Autodesk Fusion 360 part; units mm, degrees
(part 2 of 3)
sketch "Boceto7" plane through (1067.9423, 0, 0) normal (1, 0, 0) x (0, 0, -1)
  line L0 (-357.5, 27) -> (-357.5, -50.5)
  line L1 (-292.5, -50.5) -> (-292.5, 27)
  line L2 (-297.5, 22) -> (-352.5, 22)
  line L3 (-352.5, 22) -> (-352.5, -45.5)
  line L4 (-352.5, -45.5) -> (-297.5, -45.5)
  line L5 (-297.5, -11.75) -> (-352.5, -11.75) construction
  line L6 (-332.5, -16.0801) -> (-325, -20.4103)
  line L7 (-325, -20.4103) -> (-317.5, -16.0801)
  line L8 (-317.5, -16.0801) -> (-317.5, -7.4199)
  line L9 (-317.5, -7.4199) -> (-325, -3.0897)
  line L10 (-325, -3.0897) -> (-332.5, -7.4199)
  line L11 (-332.5, -7.4199) -> (-332.5, -16.0801)
  line L12 (-325, -11.75) -> (-328.75, -18.2452) construction
  line L13 (-297.5, 12.7874) -> (-302.5, 9.9006)
  line L14 (-302.5, 9.9006) -> (-302.5, 1.2404)
  line L15 (-302.5, 1.2404) -> (-297.5, -1.6464)
  line L16 (-297.5, -7.4199) -> (-305, -3.0897)
  line L17 (-305, -3.0897) -> (-312.5, -7.4199)
  line L18 (-312.5, -7.4199) -> (-312.5, -16.0801)
  line L19 (-312.5, -16.0801) -> (-305, -20.4103)
  line L20 (-305, -20.4103) -> (-297.5, -16.0801)
  line L21 (-312.5, 22) -> (-312.5, 18.5609)
  line L22 (-312.5, 18.5609) -> (-305, 14.2308)
  line L23 (-297.5, 18.5609) -> (-297.5, 22)
  line L24 (-305, 14.2308) -> (-297.5, 18.5609)
  line L25 (-307.5, 9.9006) -> (-315, 14.2308)
  line L26 (-315, 14.2308) -> (-322.5, 9.9006)
  line L27 (-322.5, 9.9006) -> (-322.5, 1.2404)
  line L28 (-322.5, 1.2404) -> (-315, -3.0897)
  line L29 (-307.5, 1.2404) -> (-307.5, 9.9006)
  line L30 (-315, -3.0897) -> (-307.5, 1.2404)
  line L31 (-332.5, 22) -> (-332.5, 18.5609)
  line L32 (-332.5, 18.5609) -> (-325, 14.2308)
  line L33 (-317.5, 18.5609) -> (-317.5, 22)
  line L34 (-325, 14.2308) -> (-317.5, 18.5609)
  line L35 (-327.5, 9.9006) -> (-335, 14.2308)
  line L36 (-335, 14.2308) -> (-342.5, 9.9006)
  line L37 (-342.5, 9.9006) -> (-342.5, 1.2404)
  line L38 (-342.5, 1.2404) -> (-335, -3.0897)
  line L39 (-327.5, 1.2404) -> (-327.5, 9.9006)
  line L40 (-335, -3.0897) -> (-327.5, 1.2404)
  line L41 (-337.5, -7.4199) -> (-345, -3.0897)
  line L42 (-345, -3.0897) -> (-352.5, -7.4199)
  line L43 (-352.5, -7.4199) -> (-352.5, -16.0801)
  line L44 (-352.5, -16.0801) -> (-345, -20.4103)
  line L45 (-337.5, -16.0801) -> (-337.5, -7.4199)
  line L46 (-345, -20.4103) -> (-337.5, -16.0801)
  line L47 (-352.5, 22) -> (-352.5, 18.5609)
  line L48 (-352.5, 18.5609) -> (-345, 14.2308)
  line L49 (-337.5, 18.5609) -> (-337.5, 22)
  line L50 (-345, 14.2308) -> (-337.5, 18.5609)
  line L51 (-347.5, 9.9006) -> (-352.5, 12.7874)
  line L52 (-347.5, 1.2404) -> (-347.5, 9.9006)
  line L53 (-352.5, -1.6464) -> (-347.5, 1.2404)
  line L54 (-297.5, -21.8536) -> (-302.5, -24.7404)
  line L55 (-302.5, -24.7404) -> (-302.5, -33.4006)
  line L56 (-297.5, -42.0609) -> (-305, -37.7308)
  line L57 (-305, -37.7308) -> (-312.5, -42.0609)
  line L58 (-312.5, -42.0609) -> (-312.5, -45.5)
  line L59 (-297.5, -45.5) -> (-297.5, -42.0609)
  line L60 (-307.5, -24.7404) -> (-315, -20.4103)
  line L61 (-315, -20.4103) -> (-322.5, -24.7404)
  line L62 (-322.5, -24.7404) -> (-322.5, -33.4006)
  line L63 (-322.5, -33.4006) -> (-315, -37.7308)
  line L64 (-307.5, -33.4006) -> (-307.5, -24.7404)
  line L65 (-315, -37.7308) -> (-307.5, -33.4006)
  line L66 (-317.5, -42.0609) -> (-325, -37.7308)
  line L67 (-325, -37.7308) -> (-332.5, -42.0609)
  line L68 (-332.5, -42.0609) -> (-332.5, -45.5)
  line L69 (-317.5, -45.5) -> (-317.5, -42.0609)
  line L70 (-327.5, -24.7404) -> (-335, -20.4103)
  line L71 (-335, -20.4103) -> (-342.5, -24.7404)
  line L72 (-342.5, -24.7404) -> (-342.5, -33.4006)
  line L73 (-342.5, -33.4006) -> (-335, -37.7308)
  line L74 (-327.5, -33.4006) -> (-327.5, -24.7404)
  line L75 (-335, -37.7308) -> (-327.5, -33.4006)
  line L76 (-337.5, -42.0609) -> (-345, -37.7308)
  line L77 (-345, -37.7308) -> (-352.5, -42.0609)
  line L78 (-352.5, -42.0609) -> (-352.5, -45.5)
  line L79 (-337.5, -45.5) -> (-337.5, -42.0609)
  line L80 (-347.5, -24.7404) -> (-352.5, -21.8536)
  line L81 (-347.5, -33.4006) -> (-347.5, -24.7404)
  line L82 (-352.5, -36.2874) -> (-347.5, -33.4006)
  line L83 (-297.5, -45.5) -> (-297.5, -42.0609)
  line L84 (-297.5, 18.5609) -> (-297.5, 22)
  line L85 (-297.5, -45.5) -> (-297.5, 22)
  line L86 (-325, -20.4103) -> (-325, -3.0897) construction
  line L87 (-297.5, -36.2874) -> (-302.5, -33.4006)
  point P0 (-325, -11.75)
  dimension "d33" = 7.5
  constraint midpoint L3 L5.end
  constraint midpoint L5 P0
  constraint parallel L3 L11
  constraint coincident P0 L12.start
  constraint midpoint L6 L12.end
  constraint coincident L4 L58.end
  constraint coincident L4 L69.start
  constraint coincident L4 L68.end
  constraint coincident L4 L79.start
  constraint coincident L3 L82.start
  constraint coincident L3 L80.end
  constraint coincident L3 L53.start
  constraint coincident L3 L51.end
  constraint coincident L2 L49.end
  constraint coincident L2 L31.start
  constraint coincident L2 L33.end
  constraint coincident L2 L21.start
  constraint collinear L83 L84
  constraint perpendicular L2 L85
  constraint symmetric L81.start L86 L55.end
  constraint symmetric L82.start L86 L87.start
  measures "d33" distance of P0 L11
extrude "Extruir5" cut sketch "Boceto7" against normal blind 240 contours L2 L21 L22 L23 L24 L84 L85 | L2 L31 L32 L33 L34 | L13 L14 L15 L85 | L2 L3 L47 L48 L49 L50 | L16 L17 L18 L19 L20 L85 | L54 L55 L85 L87 | L3 L51 L52 L53 | L4 L56 L57 L58 L59 L83 L85 | L3 L41 L42 L43 L44 L45 L46 | L3 L80 L81 L82 | L4 L66 L67 L68 L69 | L3 L4 L76 L77 L78 L79 | L6 L7 L8 L9 L10 L11 | L25 L26 L27 L28 L29 L30 | L35 L36 L37 L38 L39 L40 | L60 L61 L62 L63 L64 L65 | L70 L71 L72 L73 L74 L75 bodies 2 3
move_body "Desplazar1" bodies 1 2 3 to x (1, 0, 0) y (0, 1, 0) z (0, 0, 1) at (-888.5759, -26.6129, 0)
sketch "Boceto9" plane through (0, 0, 292.5) normal (0, 0, -1) x (-1, 0, 0)
  line L0 (0.6336, 0.3871) -> (-2.3664, 0.3871)
  line L1 (-2.3664, 0.3871) -> (-2.3664, -77.1129)
  line L2 (-2.3664, -77.1129) -> (0.6336, -77.1129)
  line L3 (0.6336, -77.1129) -> (0.6336, 0.3871)
  line L4 (0.6336, -77.1129) -> (-41.8664, -77.1129) construction
  line L5 (-41.8664, -77.1129) -> (-41.8664, -119.6129) construction
  arc A0 (-37.7625, -116.3992) -> (-2.5802, -81.2168) centre (-41.8664, -77.1129) ccw
  arc A1 (-41.8664, -119.6129) -> (0.6336, -77.1129) centre (-41.8664, -77.1129) ccw
  line L6 (0.6336, 0.3871) -> (-179.3664, 0.3871)
  line L7 (-89.3664, 0.3871) -> (-89.3664, -20) construction
  line L8 (-41.8664, -116.6129) -> (-41.8664, -119.6129)
  line L9 (0.6336, -77.1129) -> (-2.3664, -77.1129)
  line L10 (-2.3664, -77.1129) -> (-2.3664, -70.1129)
  line L11 (-2.3664, -70.1129) -> (-5.3664, -70.1129)
  line L12 (-5.3664, -70.1129) -> (-5.3664, -80.1129)
  line L13 (-5.3664, -80.1129) -> (-3.5748, -80.1129)
  line L14 (-41.8664, -116.6129) -> (-48.8664, -116.6129)
  line L15 (-48.8664, -116.6129) -> (-48.8664, -113.6129)
  line L16 (-48.8664, -113.6129) -> (-38.8664, -113.6129)
  line L17 (-38.8664, -113.6129) -> (-38.8664, -115.4046)
  arc A2 (-2.5802, -81.2168) -> (-3.5748, -80.1129) centre (-3.5748, -81.1129) ccw
  arc A3 (-38.8664, -115.4046) -> (-37.7625, -116.3992) centre (-37.8664, -115.4046) ccw
  arc A4 (-179.3664, -77.1129) -> (-136.8664, -119.6129) centre (-136.8664, -77.1129) ccw
  line L18 (-129.8664, -116.6129) -> (-129.8664, -113.6129)
  arc A5 (-176.1526, -81.2168) -> (-140.9703, -116.3992) centre (-136.8664, -77.1129) ccw
  line L19 (-136.8664, -77.1129) -> (-136.8664, -119.6129) construction
  line L20 (-136.8664, -116.6129) -> (-129.8664, -116.6129)
  arc A6 (-140.9703, -116.3992) -> (-139.8664, -115.4046) centre (-140.8664, -115.4046) ccw
  line L21 (-176.3664, -77.1129) -> (-176.3664, -70.1129)
  line L22 (-173.3664, -70.1129) -> (-173.3664, -80.1129)
  line L23 (-179.3664, -77.1129) -> (-176.3664, -77.1129)
  line L24 (-129.8664, -113.6129) -> (-139.8664, -113.6129)
  line L25 (-136.8664, -116.6129) -> (-136.8664, -119.6129)
  line L26 (-179.3664, -77.1129) -> (-136.8664, -77.1129) construction
  line L27 (-176.3664, -70.1129) -> (-173.3664, -70.1129)
  line L28 (-176.3664, -77.1129) -> (-179.3664, -77.1129)
  line L29 (-173.3664, -80.1129) -> (-175.158, -80.1129)
  line L30 (-139.8664, -113.6129) -> (-139.8664, -115.4046)
  arc A7 (-175.158, -80.1129) -> (-176.1526, -81.2168) centre (-175.158, -81.1129) ccw
  dimension "d40" = 42.5
  dimension "d41" = 42.5
  dimension "d44" = 7
  dimension "d45" = 3
  dimension "d46" = 10
  dimension "d47" = 7
  dimension "d48" = 3
  dimension "d49" = 10
  dimension "d50" = 1
  dimension "d51" = 1
  constraint coincident L2.end L3.start
  constraint perpendicular L3 L4
  constraint vertical L5
  constraint coincident L4.end L5.start
  constraint concentric A0 A1
  constraint coincident L5 L8.start
  constraint midpoint L6 L7.start
  constraint perpendicular L6 L7
  constraint coincident L1.end L2.start
  constraint perpendicular L4 L10
  constraint perpendicular L10 L11
  constraint perpendicular L11 L12
  constraint perpendicular L12 L13
  constraint perpendicular L5 L14
  constraint perpendicular L14 L15
  constraint perpendicular L15 L16
  constraint perpendicular L16 L17
  constraint tangent A0 A2
  constraint tangent L13 A2
  constraint tangent A0 A3
  constraint tangent L17 A3
  constraint symmetric L1.end L7 L21.start
  constraint symmetric L2.end L7 A4.start
  constraint symmetric L4.end L7 A4.centre
  constraint symmetric L5.end L7 A4.end
  constraint symmetric L8.start L7 L20.start
  constraint symmetric A0 L7 A5
  constraint symmetric A1 L7 A4
  constraint symmetric L7 L1.end L21.start
  constraint symmetric L7 L10.end L21.end
  constraint symmetric L7 L11.end L22.start
  constraint symmetric L7 L12.end L22.end
  constraint symmetric L7 L14.end L18.start
  constraint symmetric L7 L15.end L18.end
  constraint symmetric L7 L16.end L24.end
  constraint symmetric L7 L13.end L29.end
  constraint symmetric L7 A0.end A5.start
  constraint symmetric L7 A2 A7
  constraint symmetric L7 L17.end A6.end
  constraint symmetric L7 A0.start A5.end
  constraint symmetric L7 A3 A6
  measures "d40" distance of L2.end L4.end
  measures "d41" distance of L4.end L5.end
  measures "d44" distance of L1.end L10.end
  measures "d45" distance of L10.end L11.end
  measures "d46" distance of L11.end L12.end
  measures "d47" distance of L8.start L14.end
  measures "d48" distance of L14.end L15.end
  measures "d49" distance of L15.end L16.end
  measures "d50" radius of A2
  measures "d51" radius of A3
extrude "Extruir6" add sketch "Boceto9" against normal blind 65 separate body contours L1 L2 A0 A1 L8 L9 L10 L11 L12 L13 L14 L15 L16 L17 A2 A3 | A4 L18 A5 L20 A6 L21 L22 L23 L24 L25 L27 L28 L29 L30 A7 makes body 4 at (-0.5855, -79.1352, 335.8333) makes body 5 at (173.6725, -98.3629, 335.8333)
sketch "Boceto10" plane through (0, -116.6129, 0) normal (0, -1, 0) x (1, 0, 0)
  line L0 (129.8664, 292.5) -> (136.8664, 292.5)
  line L1 (136.8664, 292.5) -> (136.8664, 357.5)
  line L2 (136.8664, 357.5) -> (129.8664, 357.5)
  line L3 (41.8664, 292.5) -> (41.8664, 357.5)
  line L4 (136.8664, 292.5) -> (136.8664, 357.5)
  line L5 (41.8664, 357.5) -> (136.8664, 357.5)
  line L6 (136.8664, 357.5) -> (136.8664, 292.5)
  line L7 (136.8664, 292.5) -> (41.8664, 292.5)
  line L8 (41.8664, 292.5) -> (41.8664, 357.5)
  constraint horizontal L5
  constraint vertical L6
  constraint horizontal L7
  constraint vertical L8
  constraint coincident L0.end L1.start
  constraint coincident L3.end L5.start
extrude "Extruir7" add sketch "Boceto10" along normal blind 3 separate body makes body 6
sketch "Boceto11" plane through (0, -119.6129, 0) normal (0, -1, 0) x (1, 0, 0)
  line L0 (136.8664, 292.5) -> (136.8664, 357.5)
  line L1 (136.8664, 357.5) -> (41.8664, 357.5)
  line L2 (41.8664, 357.5) -> (41.8664, 292.5)
  line L3 (46.8664, 297.5) -> (131.8664, 297.5)
  line L4 (131.8664, 352.5) -> (46.8664, 352.5)
  line L5 (46.8664, 352.5) -> (46.8664, 297.5)
  line L6 (46.8664, 325) -> (131.8664, 325) construction
  line L7 (98.0267, 325) -> (93.6965, 332.5)
  line L8 (93.6965, 332.5) -> (85.0363, 332.5)
  line L9 (85.0363, 332.5) -> (80.7061, 325)
  line L10 (80.7061, 325) -> (85.0363, 317.5)
  line L11 (85.0363, 317.5) -> (93.6965, 317.5)
  line L12 (93.6965, 317.5) -> (98.0267, 325)
  line L13 (89.3664, 325) -> (89.3664, 332.5) construction
  line L14 (89.3664, 325) -> (95.8616, 328.75) construction
  line L15 (50.3953, 297.5) -> (59.0555, 297.5)
  line L16 (59.0555, 297.5) -> (63.3856, 305)
  line L17 (63.3856, 305) -> (59.0555, 312.5)
  line L18 (59.0555, 312.5) -> (50.3953, 312.5)
  line L19 (46.8664, 303.6122) -> (50.3953, 297.5)
  line L20 (50.3953, 312.5) -> (46.8664, 306.3878)
  line L21 (50.3953, 317.5) -> (59.0555, 317.5)
  line L22 (59.0555, 317.5) -> (63.3856, 325)
  line L23 (63.3856, 325) -> (59.0555, 332.5)
  line L24 (59.0555, 332.5) -> (50.3953, 332.5)
  line L25 (46.8664, 323.6122) -> (50.3953, 317.5)
  line L26 (50.3953, 332.5) -> (46.8664, 326.3878)
  line L27 (50.3953, 337.5) -> (59.0555, 337.5)
  line L28 (59.0555, 337.5) -> (63.3856, 345)
  line L29 (63.3856, 345) -> (59.0555, 352.5)
  line L30 (59.0555, 352.5) -> (50.3953, 352.5)
  line L31 (46.8664, 343.6122) -> (50.3953, 337.5)
  line L32 (50.3953, 352.5) -> (46.8664, 346.3878)
  line L33 (79.2628, 297.5) -> (76.376, 302.5)
  line L34 (76.376, 302.5) -> (67.7158, 302.5)
  line L35 (67.7158, 302.5) -> (64.829, 297.5)
  line L36 (67.7158, 307.5) -> (76.376, 307.5)
  line L37 (76.376, 307.5) -> (80.7061, 315)
  line L38 (80.7061, 315) -> (76.376, 322.5)
  line L39 (76.376, 322.5) -> (67.7158, 322.5)
  line L40 (63.3856, 315) -> (67.7158, 307.5)
  line L41 (67.7158, 322.5) -> (63.3856, 315)
  line L42 (67.7158, 327.5) -> (76.376, 327.5)
  line L43 (76.376, 327.5) -> (80.7061, 335)
  line L44 (80.7061, 335) -> (76.376, 342.5)
  line L45 (76.376, 342.5) -> (67.7158, 342.5)
  line L46 (63.3856, 335) -> (67.7158, 327.5)
  line L47 (67.7158, 342.5) -> (63.3856, 335)
  line L48 (67.7158, 347.5) -> (76.376, 347.5)
  line L49 (76.376, 347.5) -> (79.2628, 352.5)
  line L50 (64.829, 352.5) -> (67.7158, 347.5)
  line L51 (85.0363, 297.5) -> (93.6965, 297.5)
  line L52 (93.6965, 297.5) -> (98.0267, 305)
  line L53 (98.0267, 305) -> (93.6965, 312.5)
  line L54 (93.6965, 312.5) -> (85.0363, 312.5)
  line L55 (80.7061, 305) -> (85.0363, 297.5)
  line L56 (85.0363, 312.5) -> (80.7061, 305)
  line L57 (85.0363, 337.5) -> (93.6965, 337.5)
  line L58 (93.6965, 337.5) -> (98.0267, 345)
  line L59 (98.0267, 345) -> (93.6965, 352.5)
  line L60 (93.6965, 352.5) -> (85.0363, 352.5)
  line L61 (80.7061, 345) -> (85.0363, 337.5)
  line L62 (85.0363, 352.5) -> (80.7061, 345)
  line L63 (113.9038, 297.5) -> (111.017, 302.5)
  line L64 (111.017, 302.5) -> (102.3568, 302.5)
  line L65 (102.3568, 302.5) -> (99.47, 297.5)
  line L66 (102.3568, 307.5) -> (111.017, 307.5)
  line L67 (111.017, 307.5) -> (115.3472, 315)
  line L68 (115.3472, 315) -> (111.017, 322.5)
  line L69 (111.017, 322.5) -> (102.3568, 322.5)
  line L70 (98.0267, 315) -> (102.3568, 307.5)
  line L71 (102.3568, 322.5) -> (98.0267, 315)
  line L72 (102.3568, 327.5) -> (111.017, 327.5)
  line L73 (111.017, 327.5) -> (115.3472, 335)
  line L74 (115.3472, 335) -> (111.017, 342.5)
  line L75 (111.017, 342.5) -> (102.3568, 342.5)
  line L76 (98.0267, 335) -> (102.3568, 327.5)
  line L77 (102.3568, 342.5) -> (98.0267, 335)
  line L78 (102.3568, 347.5) -> (111.017, 347.5)
  line L79 (111.017, 347.5) -> (113.9038, 352.5)
  line L80 (99.47, 352.5) -> (102.3568, 347.5)
  line L81 (119.6773, 297.5) -> (128.3375, 297.5)
  line L82 (128.3375, 297.5) -> (131.8664, 303.6122)
  line L83 (131.8664, 306.3878) -> (128.3375, 312.5)
  line L84 (128.3375, 312.5) -> (119.6773, 312.5)
  line L85 (115.3472, 305) -> (119.6773, 297.5)
  line L86 (119.6773, 312.5) -> (115.3472, 305)
  line L87 (119.6773, 317.5) -> (128.3375, 317.5)
  line L88 (128.3375, 317.5) -> (131.8664, 323.6122)
  line L89 (131.8664, 326.3878) -> (128.3375, 332.5)
  line L90 (128.3375, 332.5) -> (119.6773, 332.5)
  line L91 (115.3472, 325) -> (119.6773, 317.5)
  line L92 (119.6773, 332.5) -> (115.3472, 325)
  line L93 (119.6773, 337.5) -> (128.3375, 337.5)
  line L94 (128.3375, 337.5) -> (131.8664, 343.6122)
  line L95 (131.8664, 346.3878) -> (128.3375, 352.5)
  line L96 (128.3375, 352.5) -> (119.6773, 352.5)
  line L97 (115.3472, 345) -> (119.6773, 337.5)
  line L98 (119.6773, 352.5) -> (115.3472, 345)
  line L99 (131.8664, 297.5) -> (131.8664, 303.6122)
  line L100 (131.8664, 306.3878) -> (131.8664, 352.5)
  line L101 (131.8664, 303.6122) -> (131.8664, 306.3878)
  point P0 (89.3664, 325)
  dimension "d56" = 15
  constraint midpoint L5 L6.start
  constraint midpoint L6 P0
  constraint parallel L3 L11
  constraint coincident P0 L13.start
  constraint midpoint L8 L13.end
  constraint midpoint L7 L14.end
  constraint coincident L4 L49.end
  constraint coincident L4 L50.start
  constraint coincident L4 L80.start
  constraint coincident L4 L79.end
  constraint coincident L3 L63.start
  constraint coincident L3 L65.end
  constraint coincident L3 L33.start
  constraint coincident L3 L35.end
  constraint coincident L5 L19.start
  constraint coincident L5 L20.end
  constraint coincident L5 L25.start
  constraint coincident L5 L26.end
  constraint coincident L5 L31.start
  constraint coincident L5 L32.end
  constraint coincident L89.start L99
  constraint coincident L88.end L99
  constraint coincident L94.end L99
  constraint coincident L95.start L99
  constraint collinear L99 L100
  constraint coincident L6.end L99
  measures "d56" distance of L8 L11
extrude "Extruir8" cut sketch "Boceto11" against normal blind 20 contours L3 L5 L15 L16 L17 L18 L19 L20 | L3 L33 L34 L35 | L5 L21 L22 L23 L24 L25 L26 | L3 L51 L52 L53 L54 L55 L56 | L4 L5 L27 L28 L29 L30 L31 L32 | L3 L63 L64 L65 | L3 L81 L82 L83 L84 L85 L86 L101 | L4 L48 L49 L50 | L4 L57 L58 L59 L60 L61 L62 | L87 L88 L89 L90 L91 L92 L100 | L4 L78 L79 L80 | L4 L93 L94 L95 L96 L97 L98 L100 | L7 L8 L9 L10 L11 L12 | L36 L37 L38 L39 L40 L41 | L42 L43 L44 L45 L46 L47 | L66 L67 L68 L69 L70 L71 | L72 L73 L74 L75 L76 L77 bodies 6
sketch "Boceto12" plane through (0, 0, 292.5) normal (0, 0, -1) x (-1, 0, 0)
  line L0 (0.6336, 0.3871) -> (-2.3664, 0.3871)
  line L1 (-2.3664, 0.3871) -> (-2.3664, -77.1129)
  line L2 (-2.3664, -77.1129) -> (0.6336, -77.1129)
  line L3 (0.6336, -77.1129) -> (0.6336, 0.3871)
  line L4 (-2.3664, 0.3871) -> (-2.3664, -33.6129)
  line L5 (-2.3664, -33.6129) -> (-176.3664, -33.6129)
  line L6 (-176.3664, -33.6129) -> (-176.3664, -30.6129)
  line L7 (-176.3664, -30.6129) -> (-2.3664, -30.6129)
  line L8 (-2.3664, -30.6129) -> (-2.3664, -33.6129)
  dimension "d63" = 34
  dimension "d64" = 174
  dimension "d65" = 3
  constraint vertical L4
  constraint coincident L0.end L1.start
  constraint horizontal L5
  constraint vertical L6
  constraint horizontal L7
  constraint vertical L8
  measures "d63" distance of L0.end L4.end
  measures "d64" distance of L4.end L5.end
  measures "d65" distance of L4.end L7.end
extrude "Extruir9" add sketch "Boceto12" against normal blind 62 separate body contours L1 L4 L5 L6 L7 L8 makes body 7
sketch "Boceto13" plane through (0, -33.6129, 0) normal (0, -1, 0) x (1, 0, 0)
  line L0 (2.3664, 292.5) -> (176.3664, 292.5)
  line L1 (176.3664, 292.5) -> (176.3664, 354.5)
  line L2 (176.3664, 354.5) -> (2.3664, 354.5)
  line L3 (2.3664, 354.5) -> (2.3664, 292.5)
  line L4 (2.3664, 292.5) -> (176.3664, 292.5)
  line L5 (89.3664, 292.5) -> (136.8664, 292.5)
  line L6 (89.3664, 292.5) -> (41.8664, 292.5)
  line L7 (89.3664, 296.5) -> (41.8664, 296.5)
  line L8 (89.3664, 296.5) -> (136.8664, 296.5)
  line L9 (41.8664, 296.5) -> (136.8664, 296.5)
  line L10 (136.8664, 296.5) -> (136.8664, 300.5)
  line L11 (136.8664, 300.5) -> (41.8664, 300.5)
  line L12 (41.8664, 300.5) -> (41.8664, 296.5)
  dimension "d68" = 47.5
  dimension "d69" = 47.5
  dimension "d70" = 95
  dimension "d71" = 4
  dimension "d72" = 4
  constraint coincident L0.start L3.end
  constraint coincident L0.end L1.start
  constraint midpoint L0 L5.start
  constraint parallel L0 L5
  constraint parallel L4 L6
  constraint horizontal L9
  constraint vertical L10
  constraint horizontal L11
  constraint vertical L12
  measures "d68" distance of L5.start L5.end
  measures "d69" distance of L5.start L6.end
  measures "d70" distance of L5.end L6.end
  measures "d72" distance of L7.end L11.end
extrude "Extruir10" cut sketch "Boceto13" against normal blind 5 contours L7 L8 L9 L10 L11 L12 bodies 7
sketch "Boceto14" plane through (0, 0.3871, 0) normal (0, -1, 0) x (1, 0, 0)
  line L0 (149.9882, 305) -> (154.3183, 312.5)
  line L1 (154.3183, 312.5) -> (162.9786, 312.5)
  line L2 (162.9786, 312.5) -> (167.3087, 305)
  line L3 (167.3087, 305) -> (162.9786, 297.5)
  line L4 (162.9786, 297.5) -> (154.3183, 297.5)
  line L5 (154.3183, 297.5) -> (149.9882, 305)
  line L6 (174.3664, 352.5) -> (174.3664, 347.5)
  line L7 (174.3664, 347.5) -> (171.6388, 347.5)
  line L8 (171.6388, 347.5) -> (168.7521, 352.5)
  line L9 (168.7521, 352.5) -> (174.3664, 352.5)
  line L10 (132.6677, 315) -> (136.9978, 322.5)
  line L11 (136.9978, 322.5) -> (145.6581, 322.5)
  line L12 (145.6581, 322.5) -> (149.9882, 315)
  line L13 (149.9882, 315) -> (145.6581, 307.5)
  line L14 (145.6581, 307.5) -> (136.9978, 307.5)
  line L15 (136.9978, 307.5) -> (132.6677, 315)
  line L16 (115.3472, 345) -> (119.6773, 352.5)
  line L17 (119.6773, 352.5) -> (128.3375, 352.5)
  line L18 (128.3375, 352.5) -> (132.6677, 345)
  line L19 (132.6677, 345) -> (128.3375, 337.5)
  line L20 (128.3375, 337.5) -> (119.6773, 337.5)
  line L21 (119.6773, 337.5) -> (115.3472, 345)
  line L22 (80.7061, 305) -> (85.0363, 312.5)
  line L23 (85.0363, 312.5) -> (93.6965, 312.5)
  line L24 (93.6965, 312.5) -> (98.0267, 305)
  line L25 (98.0267, 305) -> (93.6965, 297.5)
  line L26 (93.6965, 297.5) -> (85.0363, 297.5)
  line L27 (85.0363, 297.5) -> (80.7061, 305)
  line L28 (80.7061, 345) -> (85.0363, 352.5)
  line L29 (85.0363, 352.5) -> (93.6965, 352.5)
  line L30 (93.6965, 352.5) -> (98.0267, 345)
  line L31 (98.0267, 345) -> (93.6965, 337.5)
  line L32 (93.6965, 337.5) -> (85.0363, 337.5)
  line L33 (85.0363, 337.5) -> (80.7061, 345)
  line L34 (46.0651, 325) -> (50.3953, 332.5)
  line L35 (50.3953, 332.5) -> (59.0555, 332.5)
  line L36 (59.0555, 332.5) -> (63.3856, 325)
  line L37 (63.3856, 325) -> (59.0555, 317.5)
  line L38 (59.0555, 317.5) -> (50.3953, 317.5)
  line L39 (50.3953, 317.5) -> (46.0651, 325)
  line L40 (11.4241, 325) -> (15.7542, 332.5)
  line L41 (15.7542, 332.5) -> (24.4145, 332.5)
  line L42 (24.4145, 332.5) -> (28.7446, 325)
  line L43 (28.7446, 325) -> (24.4145, 317.5)
  line L44 (24.4145, 317.5) -> (15.7542, 317.5)
  line L45 (15.7542, 317.5) -> (11.4241, 325)
  line L46 (11.4241, 335) -> (7.094, 327.5)
  line L47 (7.094, 327.5) -> (4.3664, 327.5)
  line L48 (4.3664, 327.5) -> (4.3664, 342.5)
  line L49 (4.3664, 342.5) -> (7.094, 342.5)
  line L50 (7.094, 342.5) -> (11.4241, 335)
  line L51 (11.4241, 345) -> (15.7542, 352.5)
  line L52 (15.7542, 352.5) -> (24.4145, 352.5)
  line L53 (24.4145, 352.5) -> (28.7446, 345)
  line L54 (28.7446, 345) -> (24.4145, 337.5)
  line L55 (24.4145, 337.5) -> (15.7542, 337.5)
  line L56 (15.7542, 337.5) -> (11.4241, 345)
  line L57 (9.9807, 352.5) -> (7.094, 347.5)
  line L58 (7.094, 347.5) -> (4.3664, 347.5)
  line L59 (4.3664, 347.5) -> (4.3664, 352.5)
  line L60 (4.3664, 352.5) -> (9.9807, 352.5)
  line L61 (11.4241, 305) -> (15.7542, 312.5)
  line L62 (15.7542, 312.5) -> (24.4145, 312.5)
  line L63 (24.4145, 312.5) -> (28.7446, 305)
  line L64 (28.7446, 305) -> (24.4145, 297.5)
  line L65 (24.4145, 297.5) -> (15.7542, 297.5)
  line L66 (15.7542, 297.5) -> (11.4241, 305)
  line L67 (46.0651, 305) -> (50.3953, 312.5)
  line L68 (50.3953, 312.5) -> (59.0555, 312.5)
  line L69 (59.0555, 312.5) -> (63.3856, 305)
  line L70 (63.3856, 305) -> (59.0555, 297.5)
  line L71 (59.0555, 297.5) -> (50.3953, 297.5)
  line L72 (50.3953, 297.5) -> (46.0651, 305)
  line L73 (63.3856, 335) -> (67.7158, 342.5)
  line L74 (67.7158, 342.5) -> (76.376, 342.5)
  line L75 (76.376, 342.5) -> (80.7061, 335)
  line L76 (80.7061, 335) -> (76.376, 327.5)
  line L77 (76.376, 327.5) -> (67.7158, 327.5)
  line L78 (67.7158, 327.5) -> (63.3856, 335)
  line L79 (64.829, 297.5) -> (67.7158, 302.5)
  line L80 (67.7158, 302.5) -> (76.376, 302.5)
  line L81 (76.376, 302.5) -> (79.2628, 297.5)
  line L82 (79.2628, 297.5) -> (64.829, 297.5)
  line L83 (99.47, 352.5) -> (113.9038, 352.5)
  line L84 (113.9038, 352.5) -> (111.017, 347.5)
  line L85 (111.017, 347.5) -> (102.3568, 347.5)
  line L86 (102.3568, 347.5) -> (99.47, 352.5)
  line L87 (115.3472, 305) -> (119.6773, 312.5)
  line L88 (119.6773, 312.5) -> (128.3375, 312.5)
  line L89 (128.3375, 312.5) -> (132.6677, 305)
  line L90 (132.6677, 305) -> (128.3375, 297.5)
  line L91 (128.3375, 297.5) -> (119.6773, 297.5)
  line L92 (119.6773, 297.5) -> (115.3472, 305)
  line L93 (149.9882, 345) -> (154.3183, 352.5)
  line L94 (154.3183, 352.5) -> (162.9786, 352.5)
  line L95 (162.9786, 352.5) -> (167.3087, 345)
  line L96 (167.3087, 345) -> (162.9786, 337.5)
  line L97 (162.9786, 337.5) -> (154.3183, 337.5)
  line L98 (154.3183, 337.5) -> (149.9882, 345)
  line L99 (134.111, 297.5) -> (136.9978, 302.5)
  line L100 (136.9978, 302.5) -> (145.6581, 302.5)
  line L101 (145.6581, 302.5) -> (148.5448, 297.5)
  line L102 (148.5448, 297.5) -> (134.111, 297.5)
  line L103 (174.3664, 322.5) -> (174.3664, 307.5)
  line L104 (174.3664, 307.5) -> (171.6388, 307.5)
  line L105 (171.6388, 307.5) -> (167.3087, 315)
  line L106 (167.3087, 315) -> (171.6388, 322.5)
  line L107 (171.6388, 322.5) -> (174.3664, 322.5)
  line L108 (174.3664, 342.5) -> (174.3664, 327.5)
  line L109 (174.3664, 327.5) -> (171.6388, 327.5)
  line L110 (171.6388, 327.5) -> (167.3087, 335)
  line L111 (167.3087, 335) -> (171.6388, 342.5)
  line L112 (171.6388, 342.5) -> (174.3664, 342.5)
  line L113 (132.6677, 335) -> (136.9978, 342.5)
  line L114 (136.9978, 342.5) -> (145.6581, 342.5)
  line L115 (145.6581, 342.5) -> (149.9882, 335)
  line L116 (149.9882, 335) -> (145.6581, 327.5)
  line L117 (145.6581, 327.5) -> (136.9978, 327.5)
  line L118 (136.9978, 327.5) -> (132.6677, 335)
  line L119 (115.3472, 325) -> (119.6773, 332.5)
  line L120 (119.6773, 332.5) -> (128.3375, 332.5)
  line L121 (128.3375, 332.5) -> (132.6677, 325)
  line L122 (132.6677, 325) -> (128.3375, 317.5)
  line L123 (128.3375, 317.5) -> (119.6773, 317.5)
  line L124 (119.6773, 317.5) -> (115.3472, 325)
  line L125 (98.0267, 315) -> (102.3568, 322.5)
  line L126 (102.3568, 322.5) -> (111.017, 322.5)
  line L127 (111.017, 322.5) -> (115.3472, 315)
  line L128 (115.3472, 315) -> (111.017, 307.5)
  line L129 (111.017, 307.5) -> (102.3568, 307.5)
  line L130 (102.3568, 307.5) -> (98.0267, 315)
  line L131 (63.3856, 315) -> (67.7158, 322.5)
  line L132 (67.7158, 322.5) -> (76.376, 322.5)
  line L133 (76.376, 322.5) -> (80.7061, 315)
  line L134 (80.7061, 315) -> (76.376, 307.5)
  line L135 (76.376, 307.5) -> (67.7158, 307.5)
  line L136 (67.7158, 307.5) -> (63.3856, 315)
  line L137 (46.0651, 345) -> (50.3953, 352.5)
  line L138 (50.3953, 352.5) -> (59.0555, 352.5)
  line L139 (59.0555, 352.5) -> (63.3856, 345)
  line L140 (63.3856, 345) -> (59.0555, 337.5)
  line L141 (59.0555, 337.5) -> (50.3953, 337.5)
  line L142 (50.3953, 337.5) -> (46.0651, 345)
  line L143 (28.7446, 315) -> (33.0748, 322.5)
  line L144 (33.0748, 322.5) -> (41.735, 322.5)
  line L145 (41.735, 322.5) -> (46.0651, 315)
  line L146 (46.0651, 315) -> (41.735, 307.5)
  line L147 (41.735, 307.5) -> (33.0748, 307.5)
  line L148 (33.0748, 307.5) -> (28.7446, 315)
  line L149 (4.3664, 307.5) -> (4.3664, 322.5)
  line L150 (4.3664, 322.5) -> (7.094, 322.5)
  line L151 (7.094, 322.5) -> (11.4241, 315)
  line L152 (11.4241, 315) -> (7.094, 307.5)
  line L153 (7.094, 307.5) -> (4.3664, 307.5)
  line L154 (28.7446, 335) -> (33.0748, 342.5)
  line L155 (33.0748, 342.5) -> (41.735, 342.5)
  line L156 (41.735, 342.5) -> (46.0651, 335)
  line L157 (46.0651, 335) -> (41.735, 327.5)
  line L158 (41.735, 327.5) -> (33.0748, 327.5)
  line L159 (33.0748, 327.5) -> (28.7446, 335)
  line L160 (30.188, 352.5) -> (44.6218, 352.5)
  line L161 (44.6218, 352.5) -> (41.735, 347.5)
  line L162 (41.735, 347.5) -> (33.0748, 347.5)
  line L163 (33.0748, 347.5) -> (30.188, 352.5)
  line L164 (4.3664, 297.5) -> (4.3664, 302.5)
  line L165 (4.3664, 302.5) -> (7.094, 302.5)
  line L166 (7.094, 302.5) -> (9.9807, 297.5)
  line L167 (9.9807, 297.5) -> (4.3664, 297.5)
  line L168 (30.188, 297.5) -> (33.0748, 302.5)
  line L169 (33.0748, 302.5) -> (41.735, 302.5)
  line L170 (41.735, 302.5) -> (44.6218, 297.5)
  line L171 (44.6218, 297.5) -> (30.188, 297.5)
  line L172 (64.829, 352.5) -> (79.2628, 352.5)
  line L173 (79.2628, 352.5) -> (76.376, 347.5)
  line L174 (76.376, 347.5) -> (67.7158, 347.5)
  line L175 (67.7158, 347.5) -> (64.829, 352.5)
  line L176 (93.6965, 332.5) -> (98.0267, 325)
  line L177 (98.0267, 325) -> (93.6965, 317.5)
  line L178 (93.6965, 317.5) -> (85.0363, 317.5)
  line L179 (85.0363, 317.5) -> (80.7061, 325)
  line L180 (80.7061, 325) -> (85.0363, 332.5)
  line L181 (85.0363, 332.5) -> (93.6965, 332.5)
  line L182 (98.0267, 335) -> (102.3568, 342.5)
  line L183 (102.3568, 342.5) -> (111.017, 342.5)
  line L184 (111.017, 342.5) -> (115.3472, 335)
  line L185 (115.3472, 335) -> (111.017, 327.5)
  line L186 (111.017, 327.5) -> (102.3568, 327.5)
  line L187 (102.3568, 327.5) -> (98.0267, 335)
  line L188 (99.47, 297.5) -> (102.3568, 302.5)
  line L189 (102.3568, 302.5) -> (111.017, 302.5)
  line L190 (111.017, 302.5) -> (113.9038, 297.5)
  line L191 (113.9038, 297.5) -> (99.47, 297.5)
  line L192 (134.111, 352.5) -> (148.5448, 352.5)
  line L193 (148.5448, 352.5) -> (145.6581, 347.5)
  line L194 (145.6581, 347.5) -> (136.9978, 347.5)
  line L195 (136.9978, 347.5) -> (134.111, 352.5)
  line L196 (149.9882, 325) -> (154.3183, 332.5)
  line L197 (154.3183, 332.5) -> (162.9786, 332.5)
  line L198 (162.9786, 332.5) -> (167.3087, 325)
  line L199 (167.3087, 325) -> (162.9786, 317.5)
  line L200 (162.9786, 317.5) -> (154.3183, 317.5)
  line L201 (154.3183, 317.5) -> (149.9882, 325)
  line L202 (168.7521, 297.5) -> (171.6388, 302.5)
  line L203 (171.6388, 302.5) -> (174.3664, 302.5)
  line L204 (174.3664, 302.5) -> (174.3664, 297.5)
  line L205 (174.3664, 297.5) -> (168.7521, 297.5)
  line L206 (179.3664, 357.5) -> (-0.6336, 357.5)
  line L207 (-0.6336, 357.5) -> (-0.6336, 292.5)
  line L208 (-0.6336, 292.5) -> (179.3664, 292.5)
  line L209 (179.3664, 292.5) -> (179.3664, 357.5)
  line L210 (179.3664, 357.5) -> (144.3664, 357.5)
  line L211 (144.3664, 357.5) -> (144.3664, 292.5)
  line L212 (179.3664, 292.5) -> (144.3664, 292.5)
  line L213 (179.3664, 292.5) -> (179.3664, 357.5)
  line L214 (-0.6336, 357.5) -> (34.3664, 357.5)
  line L215 (34.3664, 357.5) -> (34.3664, 292.5)
  line L216 (34.3664, 292.5) -> (-0.6336, 292.5)
  line L217 (-0.6336, 292.5) -> (-0.6336, 357.5)
  dimension "d75" = 35
  dimension "d76" = 35
  dimension "d77" = 65
  constraint coincident L206.start L209.end
  constraint perpendicular L209 L210
  constraint coincident L208 L211.end
  constraint perpendicular L208 L211
  constraint coincident L208.end L209.start
  constraint horizontal L214
  constraint vertical L215
  constraint horizontal L216
  constraint vertical L217
  constraint coincident L206.end L207.start
  measures "d75" distance of L206.start L210.end
  measures "d76" distance of L206.end L214.end
  measures "d77" distance of L206.end L207.end
extrude "Extruir11" add sketch "Boceto14" against normal blind 3 contours L0 L1 L2 L3 L4 L5 | L6 L7 L8 L9 | L11 L12 L13 L14 L100 L101 L102 L114 L115 L116 L117 L192 L193 L194 L206 L208 L209 L210 L211 L212 L213 | L11 L12 L13 L14 L211 | L114 L115 L116 L117 L211 | L100 L101 L102 L211 | L192 L193 L194 L211 | L143 L144 L147 L148 L154 L155 L158 L159 L160 L162 L163 L168 L169 L171 L206 L207 L208 L214 L215 L216 L217 | L160 L162 L163 L215 | L143 L144 L147 L148 L215 | L154 L155 L158 L159 L215 | L40 L41 L42 L43 L44 L45 | L46 L47 L48 L49 L50 | L51 L52 L53 L54 L55 L56 | L57 L58 L59 L60 | L61 L62 L63 L64 L65 L66 | L93 L94 L95 L96 L97 L98 | L103 L104 L105 L106 L107 | L108 L109 L110 L111 L112 | L149 L150 L151 L152 L153 | L164 L165 L166 L167 | L196 L197 L198 L199 L200 L201 | L202 L203 L204 L205 bodies 1
sketch "Boceto15" plane through (179.3664, 0, 0) normal (1, 0, 0) x (0, 0, -1)
  line L0 (-337.5, -4.6129) -> (-337.5, -8.052)
  line L1 (-337.5, -8.052) -> (-345, -12.3822)
  line L2 (-345, -12.3822) -> (-352.5, -8.052)
  line L3 (-352.5, -8.052) -> (-352.5, -4.6129)
  line L4 (-352.5, -4.6129) -> (-337.5, -4.6129)
  line L5 (-307.5, -16.7123) -> (-307.5, -25.3725)
  line L6 (-307.5, -25.3725) -> (-315, -29.7027)
  line L7 (-315, -29.7027) -> (-322.5, -25.3725)
  line L8 (-322.5, -25.3725) -> (-322.5, -16.7123)
  line L9 (-322.5, -16.7123) -> (-315, -12.3822)
  line L10 (-315, -12.3822) -> (-307.5, -16.7123)
  line L11 (-347.5, -51.3533) -> (-347.5, -60.0136)
  line L12 (-347.5, -60.0136) -> (-352.5, -62.9003)
  line L13 (-352.5, -62.9003) -> (-352.5, -48.4666)
  line L14 (-352.5, -48.4666) -> (-347.5, -51.3533)
  line L15 (-325, -64.3437) -> (-317.5, -68.6738)
  line L16 (-317.5, -68.6738) -> (-317.5, -72.1129)
  line L17 (-317.5, -72.1129) -> (-332.5, -72.1129)
  line L18 (-332.5, -72.1129) -> (-332.5, -68.6738)
  line L19 (-332.5, -68.6738) -> (-325, -64.3437)
  line L20 (-305, -64.3437) -> (-297.5, -68.6738)
  line L21 (-297.5, -68.6738) -> (-297.5, -72.1129)
  line L22 (-297.5, -72.1129) -> (-312.5, -72.1129)
  line L23 (-312.5, -72.1129) -> (-312.5, -68.6738)
  line L24 (-312.5, -68.6738) -> (-305, -64.3437)
  line L25 (-327.5, -51.3533) -> (-327.5, -60.0136)
  line L26 (-327.5, -60.0136) -> (-335, -64.3437)
  line L27 (-335, -64.3437) -> (-342.5, -60.0136)
  line L28 (-342.5, -60.0136) -> (-342.5, -51.3533)
  line L29 (-342.5, -51.3533) -> (-335, -47.0232)
  line L30 (-335, -47.0232) -> (-327.5, -51.3533)
  line L31 (-337.5, -34.0328) -> (-337.5, -42.693)
  line L32 (-337.5, -42.693) -> (-345, -47.0232)
  line L33 (-345, -47.0232) -> (-352.5, -42.693)
  line L34 (-352.5, -42.693) -> (-352.5, -34.0328)
  line L35 (-352.5, -34.0328) -> (-345, -29.7027)
  line L36 (-345, -29.7027) -> (-337.5, -34.0328)
  line L37 (-347.5, -16.7123) -> (-347.5, -25.3725)
  line L38 (-347.5, -25.3725) -> (-352.5, -28.2593)
  line L39 (-352.5, -28.2593) -> (-352.5, -13.8255)
  line L40 (-352.5, -13.8255) -> (-347.5, -16.7123)
  line L41 (-317.5, -4.6129) -> (-317.5, -8.052)
  line L42 (-317.5, -8.052) -> (-325, -12.3822)
  line L43 (-325, -12.3822) -> (-332.5, -8.052)
  line L44 (-332.5, -8.052) -> (-332.5, -4.6129)
  line L45 (-332.5, -4.6129) -> (-317.5, -4.6129)
  line L46 (-297.5, -13.8255) -> (-297.5, -28.2593)
  line L47 (-297.5, -28.2593) -> (-302.5, -25.3725)
  line L48 (-302.5, -25.3725) -> (-302.5, -16.7123)
  line L49 (-302.5, -16.7123) -> (-297.5, -13.8255)
  line L50 (-297.5, -34.0328) -> (-297.5, -42.693)
  line L51 (-297.5, -42.693) -> (-305, -47.0232)
  line L52 (-305, -47.0232) -> (-312.5, -42.693)
  line L53 (-312.5, -42.693) -> (-312.5, -34.0328)
  line L54 (-312.5, -34.0328) -> (-305, -29.7027)
  line L55 (-305, -29.7027) -> (-297.5, -34.0328)
  line L56 (-345, -64.3437) -> (-337.5, -68.6738)
  line L57 (-337.5, -68.6738) -> (-337.5, -72.1129)
  line L58 (-337.5, -72.1129) -> (-352.5, -72.1129)
  line L59 (-352.5, -72.1129) -> (-352.5, -68.6738)
  line L60 (-352.5, -68.6738) -> (-345, -64.3437)
  line L61 (-302.5, -60.0136) -> (-302.5, -51.3533)
  line L62 (-302.5, -51.3533) -> (-297.5, -48.4666)
  line L63 (-297.5, -48.4666) -> (-297.5, -62.9003)
  line L64 (-297.5, -62.9003) -> (-302.5, -60.0136)
  line L65 (-307.5, -51.3533) -> (-307.5, -60.0136)
  line L66 (-307.5, -60.0136) -> (-315, -64.3437)
  line L67 (-315, -64.3437) -> (-322.5, -60.0136)
  line L68 (-322.5, -60.0136) -> (-322.5, -51.3533)
  line L69 (-322.5, -51.3533) -> (-315, -47.0232)
  line L70 (-315, -47.0232) -> (-307.5, -51.3533)
  line L71 (-325, -47.0232) -> (-332.5, -42.693)
  line L72 (-332.5, -42.693) -> (-332.5, -34.0328)
  line L73 (-332.5, -34.0328) -> (-325, -29.7027)
  line L74 (-325, -29.7027) -> (-317.5, -34.0328)
  line L75 (-317.5, -34.0328) -> (-317.5, -42.693)
  line L76 (-317.5, -42.693) -> (-325, -47.0232)
  line L77 (-327.5, -16.7123) -> (-327.5, -25.3725)
  line L78 (-327.5, -25.3725) -> (-335, -29.7027)
  line L79 (-335, -29.7027) -> (-342.5, -25.3725)
  line L80 (-342.5, -25.3725) -> (-342.5, -16.7123)
  line L81 (-342.5, -16.7123) -> (-335, -12.3822)
  line L82 (-335, -12.3822) -> (-327.5, -16.7123)
  line L83 (-297.5, -4.6129) -> (-297.5, -8.052)
  line L84 (-297.5, -8.052) -> (-305, -12.3822)
  line L85 (-305, -12.3822) -> (-312.5, -8.052)
  line L86 (-312.5, -8.052) -> (-312.5, -4.6129)
  line L87 (-312.5, -4.6129) -> (-297.5, -4.6129)
  line L88 (-292.5, 0.3871) -> (-357.5, 0.3871)
  line L89 (-357.5, 0.3871) -> (-357.5, -77.1129)
  line L90 (-357.5, -77.1129) -> (-292.5, -77.1129)
  line L91 (-292.5, -77.1129) -> (-292.5, 0.3871)
  line L92 (-292.5, -33.6129) -> (-354.5, -33.6129)
  line L93 (-292.5, -33.6129) -> (-292.5, -30.6129)
  line L94 (-292.5, -30.6129) -> (-354.5, -30.6129)
  line L95 (-354.5, -30.6129) -> (-354.5, -33.6129)
  line L96 (-354.5, -33.6129) -> (-292.5, -33.6129)
  line L97 (-292.5, -30.6129) -> (-292.5, -27.6129)
  line L98 (-292.5, -27.6129) -> (-357.5, -27.6129)
  line L99 (-357.5, -27.6129) -> (-357.5, -36.6129)
  line L100 (-357.5, -36.6129) -> (-292.5, -36.6129)
  line L101 (-292.5, -33.6129) -> (-292.5, -36.6129)
  line L102 (-292.5, -36.6129) -> (-292.5, -27.6129)
  dimension "d80" = 3
  dimension "d81" = 9
  constraint coincident L93.end L94.start
  constraint perpendicular L94 L97
  constraint coincident L89 L98.end
  constraint perpendicular L89 L98
  constraint perpendicular L92 L99
  constraint coincident L91 L100.end
  constraint perpendicular L91 L100
  constraint coincident L92.start L93.start
  measures "d80" distance of L93.end L97.end
  measures "d81" distance of L98.end L99.end
extrude "Extruir12" add sketch "Boceto15" against normal blind 3 contours L6 L7 L34 L35 L36 L38 L39 L46 L47 L54 L55 L73 L74 L78 L79 L89 L91 L92 L94 L95 L96 L97 L98 L99 L100 L102 | L6 L7 L98 | L46 L47 L98 | L78 L79 L98 | L38 L39 L98 | L50 L55 L91 L92 L96 L100 L101 L102 | L54 L55 L94 | L50 L53 L54 L55 L92 L96 L100 | L53 L54 L74 L75 L92 L96 L100 | L73 L74 L94 | L72 L73 L74 L75 L92 L96 L100 | L31 L34 L35 L36 L92 L96 L100 | L31 L36 L72 L73 L92 L96 L100 | L35 L36 L94 bodies 2
sketch "Boceto16" plane through (179.3664, 0, 0) normal (1, 0, 0) x (0, 0, -1)
  line L0 (-297.5, -36.6129) -> (-297.5, -42.693)
  line L1 (-297.5, -42.693) -> (-305, -47.0232)
  line L2 (-305, -47.0232) -> (-312.5, -42.693)
  line L3 (-312.5, -42.693) -> (-312.5, -36.6129)
  line L4 (-312.5, -36.6129) -> (-297.5, -36.6129)
  line L5 (-317.5, -36.6129) -> (-317.5, -42.693)
  line L6 (-317.5, -42.693) -> (-325, -47.0232)
  line L7 (-325, -47.0232) -> (-332.5, -42.693)
  line L8 (-332.5, -42.693) -> (-332.5, -36.6129)
  line L9 (-332.5, -36.6129) -> (-317.5, -36.6129)
  line L10 (-337.5, -36.6129) -> (-337.5, -42.693)
  line L11 (-337.5, -42.693) -> (-345, -47.0232)
  line L12 (-345, -47.0232) -> (-352.5, -42.693)
  line L13 (-352.5, -42.693) -> (-352.5, -36.6129)
  line L14 (-352.5, -36.6129) -> (-337.5, -36.6129)
  line L15 (-318.6195, -27.6129) -> (-322.5, -25.3725)
  line L16 (-322.5, -25.3725) -> (-322.5, -16.7123)
  line L17 (-322.5, -16.7123) -> (-315, -12.3822)
  line L18 (-315, -12.3822) -> (-307.5, -16.7123)
  line L19 (-307.5, -16.7123) -> (-307.5, -25.3725)
  line L20 (-307.5, -25.3725) -> (-311.3805, -27.6129)
  line L21 (-311.3805, -27.6129) -> (-318.6195, -27.6129)
  line L22 (-331.3805, -27.6129) -> (-338.6195, -27.6129)
  line L23 (-338.6195, -27.6129) -> (-342.5, -25.3725)
  line L24 (-342.5, -25.3725) -> (-342.5, -16.7123)
  line L25 (-342.5, -16.7123) -> (-335, -12.3822)
  line L26 (-335, -12.3822) -> (-327.5, -16.7123)
  line L27 (-327.5, -16.7123) -> (-327.5, -25.3725)
  line L28 (-327.5, -25.3725) -> (-331.3805, -27.6129)
  line L29 (-298.2272, -33.6129) -> (-311.7728, -33.6129)
  line L30 (-311.7728, -33.6129) -> (-306.5766, -30.6129)
  line L31 (-306.5766, -30.6129) -> (-303.4234, -30.6129)
  line L32 (-303.4234, -30.6129) -> (-298.2272, -33.6129)
  line L33 (-298.6195, -27.6129) -> (-302.5, -25.3725)
  line L34 (-302.5, -25.3725) -> (-302.5, -16.7123)
  line L35 (-302.5, -16.7123) -> (-297.5, -13.8255)
  line L36 (-297.5, -13.8255) -> (-297.5, -27.6129)
  line L37 (-297.5, -27.6129) -> (-298.6195, -27.6129)
  line L38 (-318.2272, -33.6129) -> (-331.7728, -33.6129)
  line L39 (-331.7728, -33.6129) -> (-326.5766, -30.6129)
  line L40 (-326.5766, -30.6129) -> (-323.4234, -30.6129)
  line L41 (-323.4234, -30.6129) -> (-318.2272, -33.6129)
  line L42 (-351.3805, -27.6129) -> (-352.5, -27.6129)
  line L43 (-352.5, -27.6129) -> (-352.5, -13.8255)
  line L44 (-352.5, -13.8255) -> (-347.5, -16.7123)
  line L45 (-347.5, -16.7123) -> (-347.5, -25.3725)
  line L46 (-347.5, -25.3725) -> (-351.3805, -27.6129)
  line L47 (-347.5, -51.3533) -> (-347.5, -60.0136)
  line L48 (-347.5, -60.0136) -> (-352.5, -62.9003)
  line L49 (-352.5, -62.9003) -> (-352.5, -48.4666)
  line L50 (-352.5, -48.4666) -> (-347.5, -51.3533)
  line L51 (-325, -64.3437) -> (-317.5, -68.6738)
  line L52 (-317.5, -68.6738) -> (-317.5, -72.1129)
  line L53 (-317.5, -72.1129) -> (-332.5, -72.1129)
  line L54 (-332.5, -72.1129) -> (-332.5, -68.6738)
  line L55 (-332.5, -68.6738) -> (-325, -64.3437)
  line L56 (-305, -64.3437) -> (-297.5, -68.6738)
  line L57 (-297.5, -68.6738) -> (-297.5, -72.1129)
  line L58 (-297.5, -72.1129) -> (-312.5, -72.1129)
  line L59 (-312.5, -72.1129) -> (-312.5, -68.6738)
  line L60 (-312.5, -68.6738) -> (-305, -64.3437)
  line L61 (-327.5, -51.3533) -> (-327.5, -60.0136)
  line L62 (-327.5, -60.0136) -> (-335, -64.3437)
  line L63 (-335, -64.3437) -> (-342.5, -60.0136)
  line L64 (-342.5, -60.0136) -> (-342.5, -51.3533)
  line L65 (-342.5, -51.3533) -> (-335, -47.0232)
  line L66 (-335, -47.0232) -> (-327.5, -51.3533)
  line L67 (-345, -64.3437) -> (-337.5, -68.6738)
  line L68 (-337.5, -68.6738) -> (-337.5, -72.1129)
  line L69 (-337.5, -72.1129) -> (-352.5, -72.1129)
  line L70 (-352.5, -72.1129) -> (-352.5, -68.6738)
  line L71 (-352.5, -68.6738) -> (-345, -64.3437)
  line L72 (-302.5, -60.0136) -> (-302.5, -51.3533)
  line L73 (-302.5, -51.3533) -> (-297.5, -48.4666)
  line L74 (-297.5, -48.4666) -> (-297.5, -62.9003)
  line L75 (-297.5, -62.9003) -> (-302.5, -60.0136)
  line L76 (-307.5, -51.3533) -> (-307.5, -60.0136)
  line L77 (-307.5, -60.0136) -> (-315, -64.3437)
  line L78 (-315, -64.3437) -> (-322.5, -60.0136)
  line L79 (-322.5, -60.0136) -> (-322.5, -51.3533)
  line L80 (-322.5, -51.3533) -> (-315, -47.0232)
  line L81 (-315, -47.0232) -> (-307.5, -51.3533)
  line L82 (-338.2272, -33.6129) -> (-351.7728, -33.6129)
  line L83 (-351.7728, -33.6129) -> (-346.5766, -30.6129)
  line L84 (-346.5766, -30.6129) -> (-343.4234, -30.6129)
  line L85 (-343.4234, -30.6129) -> (-338.2272, -33.6129)
  line L86 (-297.5, -4.6129) -> (-297.5, -8.052)
  line L87 (-297.5, -8.052) -> (-305, -12.3822)
  line L88 (-305, -12.3822) -> (-312.5, -8.052)
  line L89 (-312.5, -8.052) -> (-312.5, -4.6129)
  line L90 (-312.5, -4.6129) -> (-297.5, -4.6129)
  line L91 (-317.5, -4.6129) -> (-317.5, -8.052)
  line L92 (-317.5, -8.052) -> (-325, -12.3822)
  line L93 (-325, -12.3822) -> (-332.5, -8.052)
  line L94 (-332.5, -8.052) -> (-332.5, -4.6129)
  line L95 (-332.5, -4.6129) -> (-317.5, -4.6129)
  line L96 (-337.5, -4.6129) -> (-337.5, -8.052)
  line L97 (-337.5, -8.052) -> (-345, -12.3822)
  line L98 (-345, -12.3822) -> (-352.5, -8.052)
  line L99 (-352.5, -8.052) -> (-352.5, -4.6129)
  line L100 (-352.5, -4.6129) -> (-337.5, -4.6129)
  line L101 (-292.5, -77.1129) -> (-292.5, 0.3871)
  line L102 (-292.5, 0.3871) -> (-357.5, 0.3871)
  line L103 (-357.5, 0.3871) -> (-357.5, -77.1129)
  line L104 (-357.5, -77.1129) -> (-292.5, -77.1129)
  line L105 (-296.5, -33.6129) -> (-300.5, -33.6129)
  line L106 (-300.5, -33.6129) -> (-296.5, -33.6129)
  line L107 (-354.5, -33.6129) -> (-292.5, -33.6129)
  line L108 (-296.5, -30.6129) -> (-300.5, -30.6129)
  line L109 (-300.5, -30.6129) -> (-296.5, -30.6129)
  line L110 (-292.5, -30.6129) -> (-354.5, -30.6129)
  line L111 (-292.5, -30.6129) -> (-354.5, -30.6129)
  line L112 (-292.5, -30.6129) -> (-354.5, -30.6129)
  line L113 (-354.5, -30.6129) -> (-354.5, -33.6129)
  line L114 (-354.5, -33.6129) -> (-292.5, -33.6129)
  line L115 (-292.5, -30.6129) -> (-292.5, -33.6129)
  line L116 (-323.5, -33.6129) -> (-323.5, -36.6129) construction
  line L117 (-323.5, -33.6129) -> (-344.5, -33.6129)
  line L118 (-344.5, -33.6129) -> (-344.5, -30.6129)
  line L119 (-323.5, -33.6129) -> (-302.5, -33.6129)
  line L120 (-302.5, -33.6129) -> (-302.5, -30.6129)
  line L121 (-354.5, -33.6129) -> (-366.7409, -33.6129)
  line L122 (-366.7409, -33.6129) -> (-366.7409, -30.6129)
  line L123 (-366.7409, -30.6129) -> (-354.5, -30.6129)
  line L124 (-354.5, -30.6129) -> (-354.5, -33.6129)
  line L125 (-292.5, -33.6129) -> (-354.5, -33.6129)
  line L126 (-354.5, -30.6129) -> (-292.5, -30.6129)
  dimension "d84" = 21
  dimension "d85" = 21
  dimension "d86" = 3
  constraint coincident L110.start L111.start
  constraint coincident L110.end L111.end
  constraint coincident L107.start L113.end
  constraint coincident L107.end L114.end
  constraint midpoint L114 L116.start
  constraint coincident L9 L116.end
  constraint perpendicular L9 L116
  constraint perpendicular L113 L117
  constraint vertical L118
  constraint perpendicular L116 L119
  constraint vertical L120
  constraint coincident L110 L120.end
  constraint horizontal L121
  constraint vertical L122
  constraint horizontal L123
  constraint vertical L124
  measures "d84" distance of L116.start L117.end
  measures "d85" distance of L116.start L119.end
  measures "d86" distance of L107.start L110.end
extrude "Extruir13" cut sketch "Boceto16" against normal blind 3 contours L29 L30 L31 L32 L107 L110 L111 L112 L114 L119 L120 L125 L126 | L32 L110 L111 L112 L120 L126 | L30 L41 L107 L110 L111 L112 L114 L119 L125 L126 | L38 L39 L40 L41 L107 L110 L111 L112 L114 L117 L119 L125 L126 | L39 L85 L107 L110 L111 L112 L114 L117 L125 L126 | L82 L84 L85 L107 L110 L111 L112 L114 L117 L118 L125 L126 bodies 2
extrude "Extruir14" add sketch "Boceto16" against normal blind 3 contours L29 L32 L105 L106 L107 L114 L120 L125 | L82 L83 L84 L107 L110 L111 L112 L114 L118 L125 L126 bodies 2